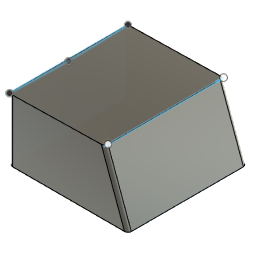
1UKeycap v2 (Autodesk Fusion 360 design; units mm, degrees)
Autodesk Fusion 360 part; units mm, degrees
sketch "Sketch1" plane through (0, 0, 0) normal (0, 0, 1) x (1, 0, 0)
  line L0 (0, 0) -> (18, 0)
  line L1 (18, 0) -> (18, 18)
  line L2 (18, 18) -> (0, 18)
  line L3 (0, 18) -> (0, 0)
  dimension "d1" = 18
  dimension "d2" = 18
  constraint horizontal L0
  constraint vertical L1
  constraint horizontal L2
  constraint vertical L3
  constraint coincident L0.start L3.end
  measures "d1" distance of L0.start L0.end
  measures "d2" distance of L0.start L2.end
sketch "Sketch2" plane through (0, 0, 0) normal (0, 1, 0) x (1, 0, 0)
  line L0 (0, 0) -> (18, 0)
  line L1 (0, 0) -> (0, -9.4)
  line L2 (18, 0) -> (28.5467, 0) construction
  line L3 (18, 0) -> (14.471, -9.6958)
  line L4 (18, 0) -> (28.318, 0) construction
  line L5 (0, -9.4) -> (14.471, -9.6958)
  dimension "d5" = 18
  dimension "d6" = 9.4
  dimension "d9" = 110
  constraint coincident L0.start L1.start
  constraint horizontal L0
  constraint perpendicular L0 L1
  constraint horizontal L2
  constraint horizontal L4
  measures "d5" distance of L0.start L0.end
  measures "d6" distance of L0.start L1.end
  measures "d9" angle of L3 L4
extrude "Extrude2" add sketch "Sketch2" along normal blind 18
shell "Shell1" thickness 1 removed faces 1 at (6, 6, 0)
sketch "Sketch3" plane through (-0.1716, 0, 8.3963) normal (0.020434, 0, -0.999791) x (0, 1, 0)
  line L0 (1, 13.9506) -> (1, 1.1718)
  line L1 (1, 1.1718) -> (17, 1.1718)
  line L2 (17, 1.1718) -> (17, 13.9506)
  line L3 (17, 13.9506) -> (1, 13.9506)
  circle A0 centre (9, 7.5612) radius 2.5
  dimension "d13" = 5
  measures "d13" diameter of A0
extrude "Extrude3" add sketch "Sketch3" along normal blind 7.5 contours A0
sketch "Sketch4" plane through (-0.0184, 0, 0.8978) normal (0.020434, 0, -0.999791) x (0, 1, 0)
  circle A0 centre (9, 7.5612) radius 2.5
  line L0 (9.55, 9.5612) -> (8.45, 9.5612)
  line L1 (8.45, 9.5612) -> (8.45, 5.5612)
  line L2 (8.45, 5.5612) -> (9.55, 5.5612)
  line L3 (9.55, 5.5612) -> (9.55, 9.5612)
  line L4 (7, 8.1862) -> (11, 8.1862)
  line L5 (11, 8.1862) -> (11, 6.9362)
  line L6 (11, 6.9362) -> (7, 6.9362)
  line L7 (7, 6.9362) -> (7, 8.1862)
  dimension "d18" = 1.1
  dimension "d19" = 4
  dimension "d22" = 4
  dimension "d23" = 1.25
  constraint horizontal L0
  constraint vertical L1
  constraint horizontal L2
  constraint vertical L3
  constraint horizontal L4
  constraint vertical L5
  constraint horizontal L6
  constraint vertical L7
  measures "d18" distance of L0.start L0.end
  measures "d19" distance of L0.start L2.end
  measures "d22" distance of L4.start L4.end
  measures "d23" distance of L4.start L6.end
extrude "Extrude4" cut sketch "Sketch4" against normal blind 8 contours L0 L1 L3 L4 | L3 L4 L5 L6 | L1 L3 L4 L6 | L1 L4 L6 L7 | L1 L2 L3 L6
fillet "Fillet1" radius 0.5 4 edges at (16.2355, 18, 4.8479) (0, 18, 4.7) (0, 0, 4.7) (16.2355, 0, 4.8479)
sketch "Sketch5" plane through (0, 0, 0) normal (-1, 0, 0) x (0, -1, 0)
  line L0 (-0.5, 0) -> (-0.5, 9.4)
  line L1 (-0.5, 9.4) -> (-17.5, 9.4)
  line L2 (-17.5, 9.4) -> (-17.5, 0)
  line L3 (-17.5, 0) -> (-0.5, 0)
  spline S0 degree 5 poles (-17.991, 9.3939) (-17.6314, 9.3724) (-16.9121, 9.3312) (-15.8333, 9.2751) (-14.3953, 9.2118) (-12.5985, 9.1532) (-10.8025, 9.117) (-9.0072, 9.105) (-7.2127, 9.1182) (-5.419, 9.1556) (-3.6261, 9.2154) (-2.1923, 9.2796) (-1.1172, 9.3365) (-0.4006, 9.3782) (-0.0423, 9.4) knots 0 0 0 0 0 0 0.1 0.2 0.3 0.4 0.5 0.6 0.7 0.8 0.9 1 1 1 1 1 1
  line L4 (-17.991, 9.3939) -> (-0.0423, 9.4)
  point P0 (-9, 9.1113)
sketch "Sketch6" plane through (15.8944, 0, 5.7851) normal (0.939693, 0, 0.34202) x (0, 1, 0)
  line L0 (0.5, 4.1616) -> (0.5, -6.1564)
  line L1 (0.5, -6.1564) -> (17.5, -6.1564)
  line L2 (17.5, -6.1564) -> (17.5, 4.1616)
  line L3 (17.5, 4.1616) -> (0.5, 4.1616)
ref_plane "WorkPlane2" through (0, 9.0167, 9.397) normal (-0.020436, 0.000337, 0.999791) x (0, -1, 0.000338)
sketch "Sketch7" plane through (0, 9.0167, 9.397) normal (-0.020436, 0.000337, 0.999791) x (0, -1, 0.000338)
  line L0 (8.5183, 14.4741) -> (9.02, 14.4741)
  line L1 (-8.4876, 14.4781) -> (-7.8669, 14.4781)
  line L2 (-7.8669, 14.4781) -> (-8.4876, 14.4781)
  line L3 (-8.9858, 14.4781) -> (9.02, 14.4741)
  constraint horizontal L0
  constraint horizontal L1
